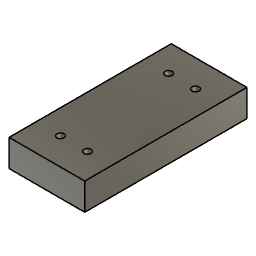
CameraOffset for long screws (Autodesk Fusion 360 design; units mm, degrees)
Autodesk Fusion 360 part; units mm, degrees
sketch "Sketch1" plane through (0, 0, 0) normal (0, 0, 1) x (1, 0, 0)
  line L0 (0, 0) -> (70, 0)
  line L1 (70, 0) -> (70, 150)
  line L2 (70, 150) -> (0, 150)
  line L3 (0, 150) -> (0, 0)
  circle A0 centre (22.5, 25) radius 3.3
  circle A1 centre (47.5, 25) radius 3.3
  circle A2 centre (22.5, 125) radius 3.3
  circle A3 centre (47.5, 125) radius 3.3
  line L4 (22.5, 25) -> (0, 25)
  line L5 (0, 25) -> (31, 25)
  line L6 (31, 25) -> (31, 37.5)
  line L7 (31, 37.5) -> (0, 37.5)
  line L8 (0, 37.5) -> (0, 25)
  line L9 (0, 25) -> (31, 25)
  line L10 (31, 25) -> (31, 12.5)
  line L11 (31, 12.5) -> (0, 12.5)
  line L12 (0, 12.5) -> (0, 25)
  line L13 (70, 37.5) -> (39, 37.5)
  line L14 (39, 37.5) -> (39, 12.5)
  line L15 (39, 12.5) -> (70, 12.5)
  line L16 (70, 12.5) -> (70, 37.5)
  line L17 (70, 137.5) -> (39, 137.5)
  line L18 (39, 137.5) -> (39, 112.5)
  line L19 (39, 112.5) -> (70, 112.5)
  line L20 (70, 112.5) -> (70, 137.5)
  line L21 (0, 137.5) -> (31, 137.5)
  line L22 (31, 137.5) -> (31, 112.5)
  line L23 (31, 112.5) -> (0, 112.5)
  line L24 (0, 112.5) -> (0, 137.5)
  point P0 (22.5, 25)
  point P1 (47.5, 25)
  point P2 (47.5, 125)
  point P3 (22.5, 125)
  dimension "d1" = 70
  dimension "d2" = 150
  dimension "d3" = 25
  dimension "d4" = 22.5
  dimension "d5" = 25
  dimension "d6" = 22.5
  dimension "d7" = 25
  dimension "d8" = 47.5
  dimension "d9" = 25
  dimension "d10" = 22.5
  dimension "d11" = 22.5
  dimension "d12" = 25
  dimension "d13" = 25
  dimension "d14" = 6.6
  dimension "d15" = 6.6
  dimension "d16" = 6.6
  dimension "d17" = 6.6
  dimension "d18" = 31
  dimension "d19" = 12.5
  dimension "d20" = 12.5
  dimension "d21" = 31
  dimension "d22" = 25
  dimension "d23" = 12.5
  dimension "d24" = 31
  dimension "d25" = 25
  dimension "d26" = 31
  dimension "d27" = 25
  dimension "d28" = 12.5
  dimension "d29" = 12.5
  constraint horizontal L0
  constraint vertical L1
  constraint horizontal L2
  constraint vertical L3
  constraint coincident L0.start L3.end
  constraint horizontal P0 P1
  constraint horizontal P2 P3
  constraint coincident P0 A0.centre
  constraint coincident P1 A1.centre
  constraint coincident P3 A2.centre
  constraint coincident P2 A3.centre
  constraint coincident L3 L4.end
  constraint perpendicular L3 L4
  constraint horizontal L5
  constraint vertical L6
  constraint horizontal L7
  constraint vertical L8
  constraint perpendicular L9 L10
  constraint parallel L9 L11
  constraint parallel L10 L12
  constraint horizontal L13
  constraint vertical L14
  constraint horizontal L15
  constraint vertical L16
  constraint coincident L1 L13.start
  constraint collinear L7 L13
  constraint horizontal L17
  constraint vertical L18
  constraint horizontal L19
  constraint vertical L20
  constraint coincident L1 L17.start
  constraint horizontal L21
  constraint vertical L22
  constraint horizontal L23
  constraint vertical L24
  constraint coincident L3 L21.start
  measures "d1" distance of L0.start L0.end
  measures "d2" distance of L0.start L2.end
  measures "d3" distance of L0 P0
  measures "d4" distance of L3 P0
  measures "d5" distance of L0 P1
  measures "d6" distance of L1 P1
  measures "d7" distance of P0 P1
  measures "d8" distance of L3 P1
  measures "d9" distance of L2 P3
  measures "d10" distance of L3 P3
  measures "d11" distance of L1 P2
  measures "d12" distance of L2 P2
  measures "d13" distance of P2 P3
  measures "d14" diameter of A0
  measures "d15" diameter of A1
  measures "d16" diameter of A2
  measures "d17" diameter of A3
  measures "d18" distance of L4.end L5.end
  measures "d19" distance of L4.end L7.end
  measures "d20" distance of L4.end L11.end
  measures "d21" distance of L13.start L13.end
  measures "d22" distance of L13.start L15.end
  measures "d23" distance of L0 L15
  measures "d24" distance of L17.start L17.end
  measures "d25" distance of L17.start L19.end
  measures "d26" distance of L21.start L21.end
  measures "d27" distance of L21.start L23.end
  measures "d28" distance of L2 L17
  measures "d29" distance of L2 L21
extrude "Extrude1" add sketch "Sketch1" along normal blind 25 contours L0 L1 L2 L3 L6 L7 L10 L11 L13 L14 L15 L17 L18 L19 L21 L22 L23 | L3 A0 L4 L5 L9 L10 L11 L12 | L1 L13 L14 L15 L16 | L3 A0 L4 L5 L6 L7 L8 L9 | L1 L17 L18 L19 L20 | L3 L21 L22 L23 L24
equation "d14 = 6 mm + 0.6 mm"
